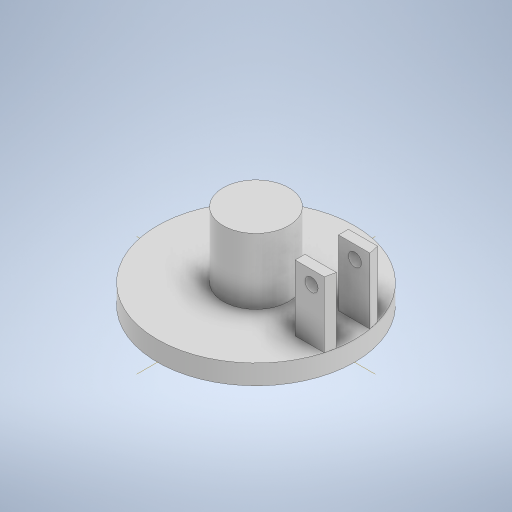
# Autodesk Inventor part: exp_latch_base_rev0
Saved by Autodesk Inventor 2024 (Build 280153000, 153)
## iProperties
Created: 2024-04-11
Part Number: exp_latch_base_rev0
Material: 一般
Document SubType Name: Modeling
Designer: Akio
Density: 1 g/cm^3
Appearance: 既定
Author: Akio
Autodesk Inventor part; units mm, degrees
ref_plane "YZ Plane" through (0, 0, 0) normal (1, 0, 0) x (0, 1, 0)
ref_plane "XZ Plane" through (0, 0, 0) normal (0, 1, 0) x (-1, 0, 0)
ref_plane "XY Plane" through (0, 0, 0) normal (0, 0, 1) x (1, 0, 0)
sketch "スケッチ1" plane through (0, 0, 0) normal (0, 1, 0) x (-1, 0, 0)
  circle A0 centre (0, 0) radius 15
  dimension "d0" = 30
  constraints: 1 centre point, 1 coincident
  measures "d0" diameter of A0
extrude "押し出し1" add sketch "スケッチ1" along normal blind 3
sketch "スケッチ2" plane through (0, 3, 0) normal (0, 1, 0) x (1, 0, 0)
  circle A0 centre (0, 0) radius 15 projected
  line L0 (14.7817, -2.55) -> (10, -2.55)
  line L1 (10, -2.55) -> (10, -4.05)
  line L2 (10, 4.05) -> (10, 2.55)
  line L3 (-21, 0) -> (21, 0) projected
  line L4 (0, 21) -> (0, -21) projected
  line L5 (10, -4.05) -> (14.4429, -4.05)
  line L6 (14.7817, -2.55) -> (14.4429, -4.05)
  line L7 (10, 2.55) -> (14.7817, 2.55)
  line L8 (10, 2.55) -> (14.7817, 2.55) construction
  line L9 (10, 4.05) -> (14.4429, 4.05)
  line L10 (14.7817, 2.55) -> (14.4429, 4.05)
  point P0 (12.3908, -2.55)
  point P1 (10, -3.3)
  point P2 (10, 3.3)
  dimension "d16" = 1.5
  dimension "d27" = 10
  dimension "d28" = 2.55
  dimension "d29" = 10
  dimension "d31" = 1.5
  dimension "d33" = 2.55
  constraints: 18 end point, 4 horizontal, 4 point on circle, 3 midpoint, 1 collinear, 1 vertical
  measures "d16" distance of L0.end L1.end
  measures "d27" distance from line of L4 point (10, -3.3)
  measures "d28" distance between parallel lines of L3 L0
  measures "d29" distance from line of L4 point (10, 3.3)
  measures "d31" distance of L2.end L2.start
  measures "d33" distance between parallel lines of L3 L7
extrude "押し出し2" add sketch "スケッチ2" along normal blind 10 contours L7 L2 L9 L10 | L6 L5 L1 L0
sketch "スケッチ4" plane through (14.4429, 3, -4.05) normal (0, 0, -1) x (-1, 0, 0)
  circle A0 centre (1.9429, 8) radius 1
  line L0 (29.4429, 0) -> (0, 0) projected
  line L1 (4.4429, 0) -> (4.4429, 10) projected
  point P0 (14.4429, -3)
  dimension "d34" = 2
  dimension "d35" = 8
  dimension "d36" = 2.5
  constraints: 1 centre point
  measures "d34" diameter of A0
  measures "d35" distance from line of L0 A0.centre
  measures "d36" distance from line of L1 A0.centre
extrude "押し出し4" cut sketch "スケッチ4" against normal through all
sketch "スケッチ5" plane through (0, 3, 0) normal (0, 1, 0) x (1, 0, 0)
  circle A0 centre (0, 0) radius 5
  dimension "d39" = 10
  constraints: 1 centre point, 1 coincident
  measures "d39" diameter of A0
extrude "押し出し5" add sketch "スケッチ5" along normal blind 10
